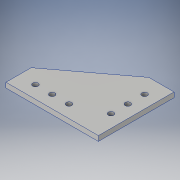
# Autodesk Inventor part: nhk24
Saved by Autodesk Inventor 2019 (Build 230136000, 136)
## iProperties
Created: 2022-02-19
Part Number: nhk24
Material: アルミニウム 6061
Document SubType Name: Sheet Metal
Designer: yuta
Density: 2.7 g/cm^3
Sheet Metal Rule: Default_mm
Appearance: アルミニウム - フラット
Author: yuta
Autodesk Inventor part; units mm, degrees
ref_plane "YZ Plane" through (0, 0, 0) normal (1, 0, 0) x (0, 1, 0)
ref_plane "XZ Plane" through (0, 0, 0) normal (0, 1, 0) x (-1, 0, 0)
ref_plane "XY Plane" through (0, 0, 0) normal (0, 0, 1) x (1, 0, 0)
sketch "スケッチ1" plane through (0, 0, 0) normal (0, 1, 0) x (-1, 0, 0)
  line L0 (9.7743, 14.6817) -> (-45.2257, 14.6817)
  line L1 (-45.2257, 14.6817) -> (-45.2257, -30.3183)
  line L2 (-45.2257, -30.3183) -> (-30.2257, -30.3183)
  line L3 (9.7743, -0.3183) -> (9.7743, 14.6817)
  line L4 (-30.2257, -30.3183) -> (9.7743, -0.3183)
  point P0 (0, 0)
  dimension "d1" = 45
  dimension "d2" = 15
  dimension "d3" = 15
  dimension "d4" = 55
  constraints: 10 end point, 2 parallel, 1 coincident, 1 horizontal, 1 perpendicular
  measures "d1" distance of L1.end L0.end
  measures "d2" distance of L3.start L0.start
  measures "d3" distance from line of L2.end L1
  measures "d4" distance of L0.start L0.end
extrude "押し出し1" add sketch "スケッチ1" along normal blind 3
sketch "スケッチ2" plane through (0, 3, 0) normal (0, 1, 0) x (1, 0, 0)
  circle A0 centre (0.2257, -7.1817) radius 1.6
  circle A1 centre (10.2257, -7.1817) radius 1.6
  circle A2 centre (20.2257, -7.1817) radius 1.6
  line L0 (45.2257, -14.6817) -> (45.2257, 30.3183) projected
  line L1 (-9.7743, -14.6817) -> (45.2257, -14.6817) projected
  circle A3 centre (37.7257, 0.3183) radius 1.6
  circle A4 centre (37.7257, 10.3183) radius 1.6
  circle A5 centre (37.7257, 20.3183) radius 1.6
  point P0 (0, 0)
  dimension "d7" = 3.2
  dimension "d8" = 3.2
  dimension "d9" = 3.2
  dimension "d10" = 25
  dimension "d11" = 45
  dimension "d12" = 35
  dimension "d13" = 7.5
  dimension "d14" = 7.5
  dimension "d15" = 7.5
  dimension "d16" = 3.2
  dimension "d17" = 7.5
  dimension "d18" = 15
  dimension "d19" = 3.2
  dimension "d20" = 10
  dimension "d21" = 3.2
  dimension "d22" = 10
  constraints: 6 centre point
  measures "d7" diameter of A0
  measures "d8" diameter of A1
  measures "d9" diameter of A2
  measures "d10" distance from line of L0 A2.centre
  measures "d11" distance from line of L0 A0.centre
  measures "d12" distance from line of L0 A1.centre
  measures "d13" distance from line of L1 A0.centre
  measures "d14" distance from line of L1 A1.centre
  measures "d15" distance from line of L1 A2.centre
  measures "d16" diameter of A3
  measures "d17" distance from line of L0 A3.centre
  measures "d18" distance from line of L1 A3.centre
  measures "d19" diameter of A4
  measures "d20" distance of A4.centre A3.centre
  measures "d21" diameter of A5
  measures "d22" distance of A4.centre A5.centre
hole "穴1" at (0.2257, 3, 7.1817) at (10.2257, 3, 7.1817) at (20.2257, 3, 7.1817) at (37.7257, 3, -0.3183) at (37.7257, 3, -10.3183) at (37.7257, 3, -20.3183) direction (0, -1, 0) diameter 3.2 depth 3
equation "\"BendRadius\" = Thickness"
equation "\"BendReliefWidth\" = Thickness"
equation "\"BendReliefDepth\" = 0.5 * Thickness"
equation "\"CornerReliefSize\" = 4 * Thickness"
equation "\"MinimumRemnant\" = 2 * Thickness"
equation "\"TransitionRadius\" = BendRadius"
equation "\"JacobiRadiusSize\" = BendRadius"
equation "\"GapSize\" = Thickness"
equation "\"Thickness\" = 0.5"
